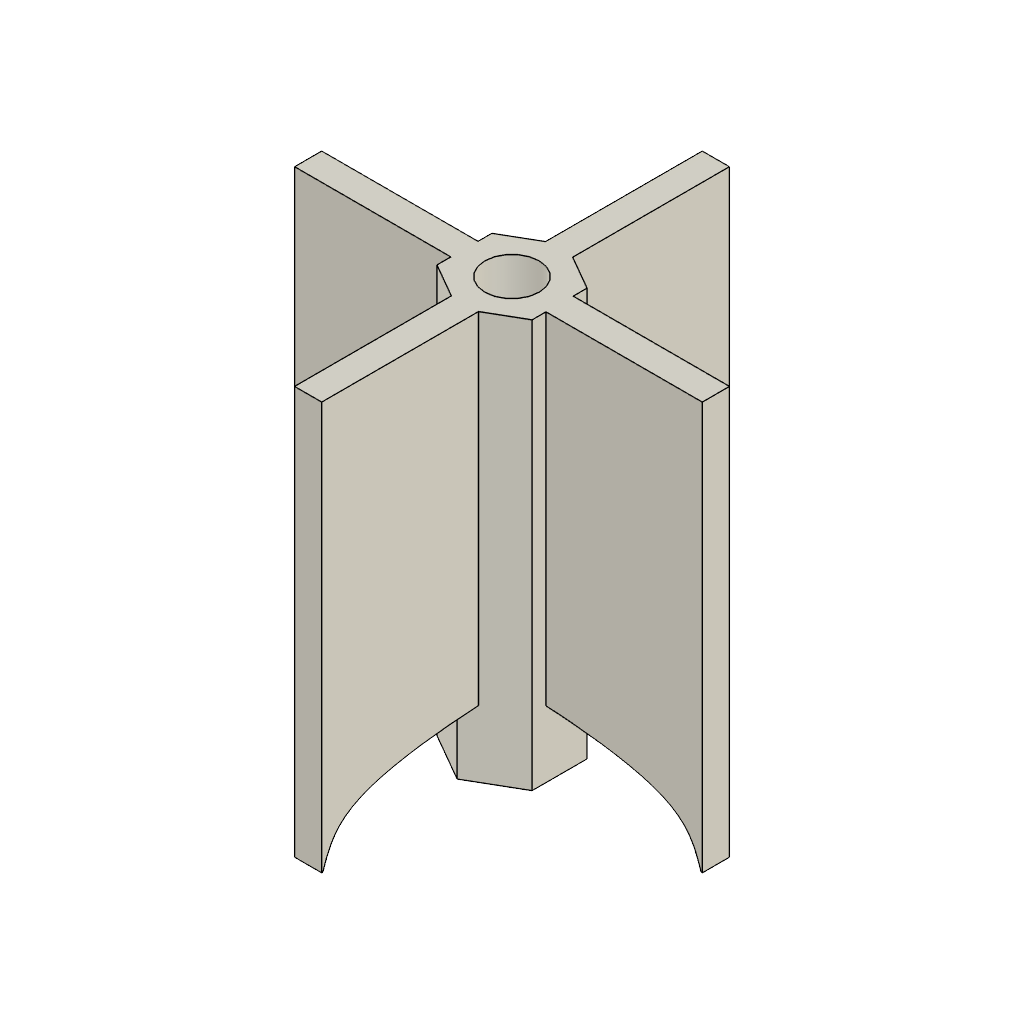
Sensor Assembly (Autodesk Fusion 360 archive; units mm, degrees)
design "Sensor Divider 3 cm"
part number: 2026-09-18-10-50-11-663
Autodesk Fusion 360 part; units mm, degrees
sketch "Sketch1" plane through (0, 0, 0) normal (0, 0, 1) x (1, 0, 0)
  line L0 (-15, 0) -> (15, 0)
  line L1 (0, -15) -> (0, 15)
  line L2 (1, 15) -> (-1, 15)
  line L3 (-1, 15) -> (-1, -15)
  line L4 (-1, -15) -> (1, -15)
  line L5 (1, -15) -> (1, 15)
  line L6 (1, 15) -> (-1, -15) construction
  line L7 (-1, 15) -> (1, -15) construction
  line L8 (15, -1) -> (-15, -1)
  line L9 (-15, -1) -> (-15, 1)
  line L10 (-15, 1) -> (15, 1)
  line L11 (15, 1) -> (15, -1)
  line L12 (15, -1) -> (-15, 1) construction
  line L13 (-15, -1) -> (15, 1) construction
  line L14 (3.5, 2.25) -> (3.5, -2.25)
  line L15 (-0.1986, -4.1561) -> (3.6986, -1.9061)
  line L16 (0.1986, -4.1561) -> (-3.6986, -1.9061)
  line L17 (-3.6986, 1.9061) -> (0.1986, 4.1561)
  line L18 (3.6986, 1.9061) -> (-0.1986, 4.1561)
  line L19 (-3.5, 2.25) -> (-3.5, -2.25)
  circle A0 centre (0, 0) radius 2
  dimension "d1" = 30
  dimension "d2" = 30
  dimension "d3" = 4.5
  dimension "d4" = 4.5
  dimension "d5" = 4
  constraint midpoint L0 A0.centre
  constraint coincident A0.centre origin
  constraint horizontal L0
  constraint midpoint L1 A0.centre
  constraint perpendicular L0 L1
  constraint horizontal L2
  constraint perpendicular L2 L3
  constraint parallel L2 L4
  constraint parallel L3 L5
  constraint coincident L6 A0.centre
  constraint coincident L7 A0.centre
  constraint horizontal L8
  constraint perpendicular L8 L9
  constraint parallel L8 L10
  constraint parallel L9 L11
  constraint coincident L12 A0.centre
  constraint coincident L13 A0.centre
  measures "d1" distance of L0.start L0.end
  measures "d2" distance of L1.start L1.end
  measures "d3" distance of L14.start L14.end
  measures "d4" distance of L19.start L19.end
  measures "d5" diameter of A0
extrude "Extrude1" add sketch "Sketch1" along normal blind 30 contours L0 L9 L10 L19 | L0 L8 L9 L19 | L0 L10 L19 A0 | L0 L8 L19 A0 | L3 L10 L17 L19 A0 | L3 L8 L16 L19 A0 | L1 L3 L17 A0 | L1 L3 L16 A0 | L1 L2 L3 L17 | L1 L3 L4 L16 | L1 L5 L18 A0 | L1 L5 L15 A0 | L1 L2 L5 L18 | L1 L4 L5 L15 | L0 L10 L14 A0 | L0 L8 L14 A0 | L5 L10 L14 L18 A0 | L5 L8 L14 L15 A0 | L0 L10 L11 L14 | L0 L8 L11 L14
sketch "Sketch2" plane through (0, 0, 0) normal (0, 1, 0) x (1, 0, 0)
  spline S0 degree 5 poles (1.976, -4.9412) (2.1036, -4.9412) (2.3816, -4.9392) (2.8674, -4.93) (3.6828, -4.9007) (5.1251, -4.8061) (7.0462, -4.6109) (9.3872, -4.2698) (11.6257, -3.7307) (13.1893, -2.974) (14.1339, -2.0321) (14.549, -1.1666) (14.7949, -0.4741) (14.9482, 0.0041) (15.0223, 0.2474) knots 0 0 0 0 0 0 0.1 0.2 0.3 0.4 0.5 0.6 0.7 0.8 0.9 1 1 1 1 1 1
  line L0 (1.3362, -4.9412) -> (2.6158, -4.9412)
  line L1 (7.3223, -4.6412) -> (11.7829, -3.7228)
  line L2 (14.6638, -0.9298) -> (15.3808, 1.4246)
  line L3 (15.0223, -4.9412) -> (15.0223, 0.2474)
  line L4 (1.976, -4.9412) -> (15.0223, -4.9412)
  line L5 (15.0223, 0.2474) -> (1.976, 0.2474)
  line L6 (1.976, 0.2474) -> (1.976, -4.9412)
  line L7 (0, 0) -> (0, -4)
  point P0 (9.5526, -4.182)
  constraint midpoint P0 L1
  constraint midpoint S0.end L2
  constraint midpoint S0.start L0
  constraint coincident L0.end L4
  constraint coincident L7.start origin
  constraint vertical L7
revolve "Revolve1" cut sketch "Sketch2" angle 360 about axis through (0, 0, 0) along (0, 0, 1) contours S0 L5 L6
sketch "Sketch3" plane through (0, 0, 0) normal (0, 0, 1) x (1, 0, 0)
  line L0 (3.6986, 1.9061) -> (-0.1986, 4.1561)
  line L1 (-0.1986, -4.1561) -> (3.6986, -1.9061)
  line L2 (0.1986, -4.1561) -> (-3.6986, -1.9061)
  line L3 (-3.6986, 1.9061) -> (0.1986, 4.1561)
  line L4 (-3.5, 2.25) -> (-3.5, -2.25)
  line L5 (3.5, 2.25) -> (3.5, -2.25)
  dimension "d9" = 4.5
  dimension "d10" = 4.5
  measures "d9" distance of L5.start L5.end
  measures "d10" distance of L4.start L4.end
sketch "Sketch4" plane through (0, 0, 0) normal (0, 0, 1) x (1, 0, 0)
extrude "Extrude2" add sketch "Sketch3" along normal blind 9.5
sketch "Sketch5" plane through (0, 0, 0) normal (0, 0, -1) x (1, 0, 0)
  line L0 (3.5, 2.0207) -> (0, 4.0415)
  line L1 (0, 4.0415) -> (-3.5, 2.0207)
  line L2 (-3.5, 2.0207) -> (-3.5, -2.0207)
  line L3 (-3.5, -2.0207) -> (0, -4.0415)
  line L4 (0, -4.0415) -> (3.5, -2.0207)
  line L5 (3.5, -2.0207) -> (3.5, 2.0207)
  circle A0 centre (0, 0) radius 2
  dimension "d13" = 4
  constraint coincident A0.centre origin
  measures "d13" diameter of A0
extrude "Extrude3" cut sketch "Sketch5" against normal blind 28.5 contours A0

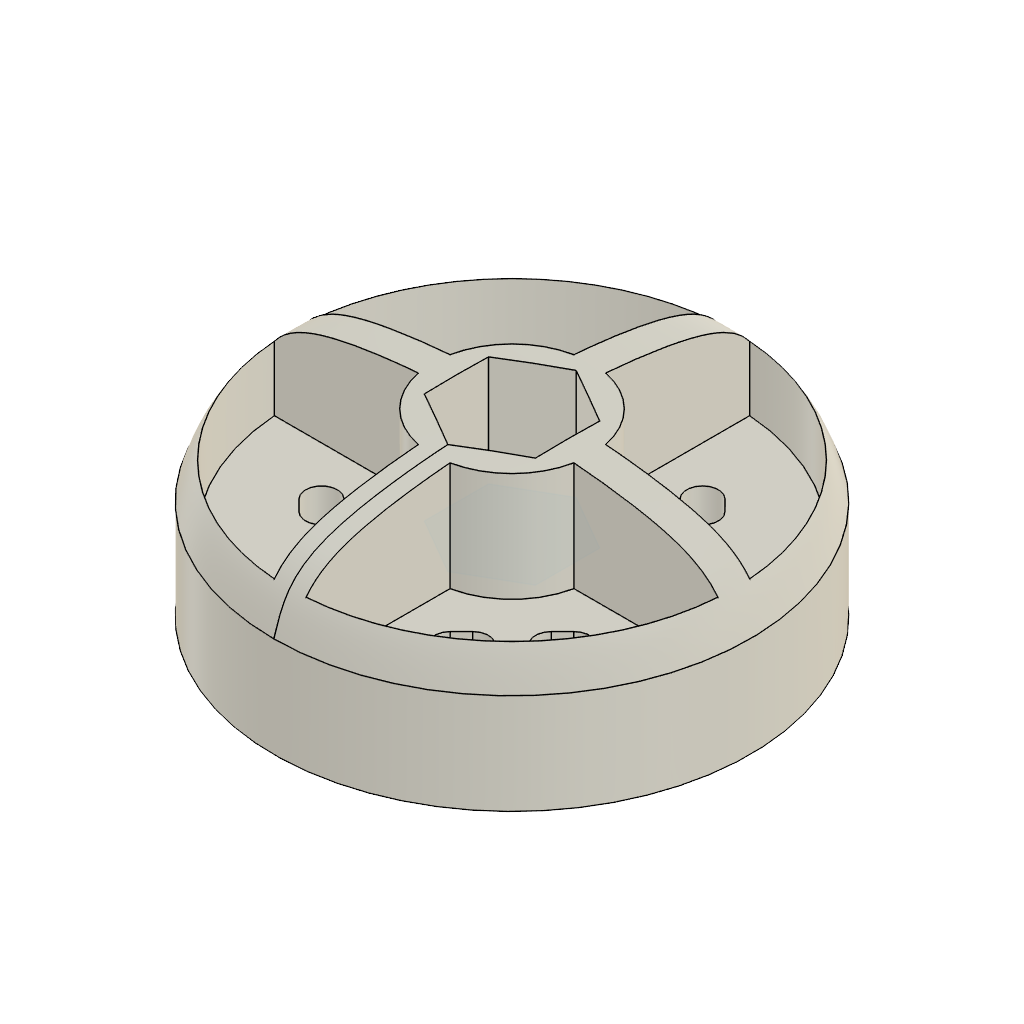
design "Sensor case Top V2"
part number: 2026-09-12-18-50-55-083
Autodesk Fusion 360 part; units mm, degrees
sketch "Sketch1" plane through (0, 0, 0) normal (0, 0, 1) x (1, 0, 0)
  circle A0 centre (0, 0) radius 15
  line L0 (-3.3472, 7.2366) -> (-4.0543, 6.5295)
  arc A1 (-3.3472, 7.2366) -> (-4.7617, 8.6505) centre (-4.0543, 7.9437) ccw
  arc A2 (-5.4683, 7.944) -> (-4.0543, 6.5295) centre (-4.7614, 7.2366) ccw
  line L1 (-4.7614, 8.6508) -> (-5.4685, 7.9437)
  arc A3 (-6.5292, 4.0546) -> (-7.963, 5.4487) centre (-7.2363, 4.7617) ccw
  line L2 (-7.963, 5.4487) -> (-8.6502, 4.762)
  arc A4 (-8.6502, 4.762) -> (-7.2363, 3.3475) centre (-7.9434, 4.0546) ccw
  line L3 (-6.5292, 4.0546) -> (-7.2363, 3.3475)
  line L4 (0, 15) -> (0, -15)
  line L5 (-15, 0) -> (15, 0)
  line L6 (0, 0) -> (-6, 6)
  line L7 (-4.7614, 7.2366) -> (-7.2363, 4.7617)
  circle A5 centre (-5.9989, 5.9992) radius 0.2772
  arc A6 (-7.944, -5.4683) -> (-6.5295, -4.0543) centre (-7.2366, -4.7614) ccw
  line L8 (-7.2366, -3.3472) -> (-6.5295, -4.0543)
  arc A7 (-7.2366, -3.3472) -> (-8.6505, -4.7617) centre (-7.9437, -4.0543) ccw
  line L9 (-8.6508, -4.7614) -> (-7.9437, -5.4685)
  arc A8 (-4.0546, -6.5292) -> (-5.4487, -7.963) centre (-4.7617, -7.2363) ccw
  line L10 (-5.4487, -7.963) -> (-4.762, -8.6502)
  arc A9 (-4.762, -8.6502) -> (-3.3475, -7.2363) centre (-4.0546, -7.9434) ccw
  line L11 (-4.0546, -6.5292) -> (-3.3475, -7.2363)
  arc A10 (5.4683, -7.944) -> (4.0543, -6.5295) centre (4.7614, -7.2366) ccw
  line L12 (3.3472, -7.2366) -> (4.0543, -6.5295)
  arc A11 (3.3472, -7.2366) -> (4.7617, -8.6505) centre (4.0543, -7.9437) ccw
  line L13 (4.7614, -8.6508) -> (5.4685, -7.9437)
  arc A12 (6.5292, -4.0546) -> (7.963, -5.4487) centre (7.2363, -4.7617) ccw
  line L14 (7.963, -5.4487) -> (8.6502, -4.762)
  arc A13 (8.6502, -4.762) -> (7.2363, -3.3475) centre (7.9434, -4.0546) ccw
  line L15 (6.5292, -4.0546) -> (7.2363, -3.3475)
  arc A14 (7.944, 5.4683) -> (6.5295, 4.0543) centre (7.2366, 4.7614) ccw
  line L16 (7.2366, 3.3472) -> (6.5295, 4.0543)
  arc A15 (7.2366, 3.3472) -> (8.6505, 4.7617) centre (7.9437, 4.0543) ccw
  line L17 (8.6508, 4.7614) -> (7.9437, 5.4685)
  arc A16 (4.0546, 6.5292) -> (5.4487, 7.963) centre (4.7617, 7.2363) ccw
  line L18 (5.4487, 7.963) -> (4.762, 8.6502)
  arc A17 (4.762, 8.6502) -> (3.3475, 7.2363) centre (4.0546, 7.9434) ccw
  line L19 (4.0546, 6.5292) -> (3.3475, 7.2363)
  dimension "d1" = 30
  dimension "d29" = 2
  dimension "d30" = 2
  dimension "d31" = 2
  dimension "d32" = 2
  dimension "d34" = 360
  constraint coincident A0.centre L6.start
  constraint coincident L2.end A4
  constraint tangent L2 A4
  constraint tangent A4 L3
  constraint coincident A4.start L2
  constraint coincident A1.end L1
  constraint coincident A2.start L1
  constraint coincident A0 L4.start
  constraint coincident A0 L4.end
  constraint perpendicular A0 L4
  constraint coincident A0 L5.start
  constraint coincident A0 L5.end
  constraint perpendicular A0 L5
  constraint coincident A2.centre L7.start
  constraint coincident A3.centre L7.end
  constraint midpoint L7 A5.centre
  measures "d1" diameter of A0
  measures "d29" diameter of A3
  measures "d30" diameter of A2
  measures "d31" diameter of A4
  measures "d32" diameter of A1
extrude "Extrude1" add sketch "Sketch1" along normal blind 4.5 contours A0 L4 L5 | A0 L4 L5 | A0 L4 L5 | A0 L4 L5 | L6 L7 A5 | L6 L7 A5 | L7 A5
sketch "Sketch2" plane through (0, 0, 4.5) normal (0, 0, 1) x (-1, 0, 0)
  circle A0 centre (0, 0) radius 15
  line L0 (8.6502, -4.762) -> (7.963, -5.4487)
  arc A1 (6.5292, -4.0546) -> (7.963, -5.4487) centre (7.2363, -4.7617) ccw
  line L1 (6.5292, -4.0546) -> (7.2363, -3.3475)
  arc A2 (8.6502, -4.762) -> (7.2363, -3.3475) centre (7.9434, -4.0546) ccw
  line L2 (-8.6502, 4.762) -> (-7.963, 5.4487)
  arc A3 (-6.5292, 4.0546) -> (-7.963, 5.4487) centre (-7.2363, 4.7617) ccw
  line L3 (-6.5292, 4.0546) -> (-7.2363, 3.3475)
  arc A4 (-8.6502, 4.762) -> (-7.2363, 3.3475) centre (-7.9434, 4.0546) ccw
  arc A5 (3.3472, -7.2366) -> (4.7614, -8.6508) centre (4.0543, -7.9437) ccw
  line L4 (3.3472, -7.2366) -> (4.0543, -6.5295)
  arc A6 (5.4685, -7.9437) -> (4.0543, -6.5295) centre (4.7614, -7.2366) ccw
  line L5 (5.4685, -7.9437) -> (4.7614, -8.6508)
  line L6 (-4.762, -8.6502) -> (-5.4487, -7.963)
  arc A7 (-4.0546, -6.5292) -> (-5.4487, -7.963) centre (-4.7617, -7.2363) ccw
  line L7 (-4.0546, -6.5292) -> (-3.3475, -7.2363)
  arc A8 (-4.762, -8.6502) -> (-3.3475, -7.2363) centre (-4.0546, -7.9434) ccw
  arc A9 (7.2366, 3.3472) -> (8.6508, 4.7614) centre (7.9437, 4.0543) ccw
  line L8 (7.2366, 3.3472) -> (6.5295, 4.0543)
  arc A10 (7.9437, 5.4685) -> (6.5295, 4.0543) centre (7.2366, 4.7614) ccw
  line L9 (7.9437, 5.4685) -> (8.6508, 4.7614)
  line L10 (4.762, 8.6502) -> (5.4487, 7.963)
  arc A11 (4.0546, 6.5292) -> (5.4487, 7.963) centre (4.7617, 7.2363) ccw
  line L11 (4.0546, 6.5292) -> (3.3475, 7.2363)
  arc A12 (4.762, 8.6502) -> (3.3475, 7.2363) centre (4.0546, 7.9434) ccw
  arc A13 (-7.2366, -3.3472) -> (-8.6508, -4.7614) centre (-7.9437, -4.0543) ccw
  line L12 (-7.2366, -3.3472) -> (-6.5295, -4.0543)
  arc A14 (-7.9437, -5.4685) -> (-6.5295, -4.0543) centre (-7.2366, -4.7614) ccw
  line L13 (-7.9437, -5.4685) -> (-8.6508, -4.7614)
  arc A15 (-3.3472, 7.2366) -> (-4.7614, 8.6508) centre (-4.0543, 7.9437) ccw
  line L14 (-3.3472, 7.2366) -> (-4.0543, 6.5295)
  arc A16 (-5.4685, 7.9437) -> (-4.0543, 6.5295) centre (-4.7614, 7.2366) ccw
  line L15 (-5.4685, 7.9437) -> (-4.7614, 8.6508)
  line L16 (0, 0) -> (0, -15)
  line L17 (0, 15) -> (0, 0)
  line L18 (15, 0) -> (-15, 0)
  circle A17 centre (0, 0) radius 14
  line L19 (-1, -15) -> (1, -15)
  line L20 (1, -15) -> (1, 15)
  line L21 (1, 15) -> (-1, 15)
  line L22 (-1, 15) -> (-1, -15)
  line L23 (-1, -15) -> (1, 15) construction
  line L24 (1, -15) -> (-1, 15) construction
  line L25 (-15, 1) -> (15, 1)
  line L26 (15, 1) -> (15, -1)
  line L27 (15, -1) -> (-15, -1)
  line L28 (-15, -1) -> (-15, 1)
  line L29 (-15, 1) -> (15, -1) construction
  line L30 (15, 1) -> (-15, -1) construction
  line L31 (3.5, 0) -> (-3.5, 0)
  circle A18 centre (6, -6) radius 2.5
  line L32 (3.5, 2.25) -> (3.5, -2.25)
  line L33 (-3.5, 2.25) -> (-3.5, -2.25)
  line L34 (-3.6986, 1.9061) -> (0.1986, 4.1561)
  line L35 (-0.1986, -4.1561) -> (3.6986, -1.9061)
  line L36 (0.1986, -4.1561) -> (-3.6986, -1.9061)
  line L37 (3.6986, 1.9061) -> (-0.1986, 4.1561)
  circle A19 centre (0, 0) radius 5
  dimension "d37" = 28
  dimension "d38" = 7
  dimension "d39" = 5
  dimension "d40" = 4.5
  dimension "d41" = 4.5
  dimension "d43" = 360
  dimension "d44" = 10
  constraint coincident A0.centre L16.start
  constraint coincident A0 L16.end
  constraint vertical L16
  constraint coincident A0 L17.start
  constraint parallel L16 L17
  constraint coincident A0 L18.start
  constraint coincident A0 L18.end
  constraint perpendicular A0 L18
  constraint horizontal L19
  constraint perpendicular L19 L20
  constraint parallel L19 L21
  constraint parallel L20 L22
  constraint coincident L23 A0.centre
  constraint coincident L24 A0.centre
  constraint horizontal L25
  constraint perpendicular L25 L26
  constraint parallel L25 L27
  constraint parallel L26 L28
  constraint coincident L29 A0.centre
  constraint coincident L30 A0.centre
  constraint midpoint A0.centre L31
  constraint perpendicular L16 L31
  constraint midpoint L31.start L32
  constraint perpendicular L27 L32
  constraint midpoint L31.end L33
  constraint perpendicular L27 L33
  measures "d37" diameter of A17
  measures "d38" distance of L31.start L31.end
  measures "d39" diameter of A18
  measures "d40" distance of L32.start L32.end
  measures "d41" distance of L33.start L33.end
  measures "d44" diameter of A19
extrude "Extrude2" add sketch "Sketch2" along normal blind 7 contours A0 L18 A17 L25 | A0 L18 A17 L27 | A0 A17 L20 L25 | A0 A17 L20 L27 | L18 A17 L27 A19 | L18 A17 L25 A19 | A0 L17 A17 L20 | A0 L16 A17 L20 | L18 L27 L32 A19 | L18 L25 L32 A19 | A0 L17 A17 L22 | L17 A17 L20 A19 | L20 L25 L32 L37 A19 | A0 L16 A17 L22 | L16 A17 L20 A19 | L20 L27 L32 L35 A19 | A0 A17 L22 L25 | L17 A17 L22 A19 | L17 L20 L37 A19 | A0 A17 L22 L27 | L16 A17 L22 A19 | L16 L20 L35 A19 | A0 L18 A17 L25 | L17 L22 L34 A19 | A0 L18 A17 L27 | L16 L22 L36 A19 | L18 A17 L25 A19 | L22 L25 L33 L34 A19 | L18 A17 L27 A19 | L22 L27 L33 L36 A19 | L18 L25 L33 A19 | L18 L27 L33 A19
sketch "Sketch3" plane through (0, 0, 0) normal (1, 0, 0) x (0, 1, 0)
  spline S0 degree 5 poles (-1.9536, 11.5) (-2.0813, 11.5) (-2.3593, 11.498) (-2.8451, 11.4888) (-3.6605, 11.4595) (-5.1028, 11.3649) (-7.0239, 11.1697) (-9.3649, 10.8286) (-11.6033, 10.2895) (-13.167, 9.5328) (-14.1116, 8.5909) (-14.5267, 7.7254) (-14.7726, 7.0329) (-14.9259, 6.5546) (-15, 6.3114) knots 0 0 0 0 0 0 0.1 0.2 0.3 0.4 0.5 0.6 0.7 0.8 0.9 1 1 1 1 1 1
  line L0 (-1.9536, 11.5) -> (-15, 11.5)
  line L1 (-15, 11.5) -> (-15, 6.3114)
  line L2 (-15, 6.3114) -> (-1.9536, 6.3114)
  line L3 (-1.9536, 6.3114) -> (-1.9536, 11.5)
  line L4 (-7.3, 11.2) -> (-11.7606, 10.2816)
  line L5 (-14.6415, 7.4886) -> (-15.3585, 5.1342)
  line L6 (0, 10) -> (0, 15)
  line L7 (-1.3138, 11.5) -> (-2.5934, 11.5)
  point P0 (-9.5303, 10.7408)
  constraint horizontal L0
  constraint vertical L1
  constraint horizontal L2
  constraint vertical L3
  constraint midpoint P0 L4
  constraint midpoint S0.end L5
  constraint vertical L6
  constraint midpoint S0.start L7
  constraint coincident L0 L7.end
revolve "Revolve1" cut sketch "Sketch3" angle 360 about axis through (0, 0, 10) along (0, 0, 1) contours S0 L0 L1 L7
sketch "Sketch4" plane through (0, 0, 4.5) normal (0, 0, 1) x (-1, 0, 0)
  line L0 (-3.5, -2.0207) -> (0, -4.0415)
  line L1 (0, -4.0415) -> (3.5, -2.0207)
  line L2 (3.5, -2.0207) -> (3.5, 2.0207)
  line L3 (3.5, 2.0207) -> (0, 4.0415)
  line L4 (0, 4.0415) -> (-3.5, 2.0207)
  line L5 (-3.5, 2.0207) -> (-3.5, -2.0207)
sketch "Sketch5" plane through (0, 0, 4.5) normal (0, 0, 1) x (-1, 0, 0)
  circle A0 centre (0, 0) radius 2
  dimension "d48" = 4
  constraint coincident A0.centre origin
  measures "d48" diameter of A0
extrude "Extrude3" cut sketch "Sketch5" against normal blind 17
sketch "Sketch6" plane through (0, 0, 4.5) normal (0, 0, 1) x (-1, 0, 0)
  line L0 (13.9642, -1) -> (4.899, -1)
  arc A0 (1, -4.899) -> (4.899, -1) centre (0, 0) ccw
  line L1 (1, -4.899) -> (1, -13.9642)
  arc A1 (1, -13.9642) -> (13.9642, -1) centre (0, 0) ccw
  arc A2 (3.3472, -7.2366) -> (4.7614, -8.6508) centre (4.0543, -7.9437) ccw
  line L2 (3.3472, -7.2366) -> (4.0543, -6.5295)
  arc A3 (5.4685, -7.9437) -> (4.0543, -6.5295) centre (4.7614, -7.2366) ccw
  line L3 (5.4685, -7.9437) -> (4.7614, -8.6508)
  line L4 (8.6502, -4.762) -> (7.963, -5.4487)
  arc A4 (6.5292, -4.0546) -> (7.963, -5.4487) centre (7.2363, -4.7617) ccw
  line L5 (6.5292, -4.0546) -> (7.2363, -3.3475)
  arc A5 (8.6502, -4.762) -> (7.2363, -3.3475) centre (7.9434, -4.0546) ccw
  line L6 (7.2363, -4.7617) -> (4.7614, -7.2366)
  line L7 (6.8082, -4.8211) -> (4.8333, -6.8263)
  line L8 (4.8333, -6.8263) -> (5.1895, -7.1772)
  line L9 (5.1895, -7.1772) -> (7.1645, -5.172)
  line L10 (7.1645, -5.172) -> (6.8082, -4.8211)
  line L11 (6.8082, -4.8211) -> (5.1895, -7.1772) construction
  line L12 (4.8333, -6.8263) -> (7.1645, -5.172) construction
  line L13 (6.8263, 4.8333) -> (7.1772, 5.1895)
  line L14 (7.1772, 5.1895) -> (5.172, 7.1645)
  line L15 (4.8211, 6.8082) -> (6.8263, 4.8333)
  line L16 (5.172, 7.1645) -> (4.8211, 6.8082)
  line L17 (-4.8333, 6.8263) -> (-5.1895, 7.1772)
  line L18 (-5.1895, 7.1772) -> (-7.1645, 5.172)
  line L19 (-6.8082, 4.8211) -> (-4.8333, 6.8263)
  line L20 (-7.1645, 5.172) -> (-6.8082, 4.8211)
  line L21 (-6.8263, -4.8333) -> (-7.1772, -5.1895)
  line L22 (-7.1772, -5.1895) -> (-5.172, -7.1645)
  line L23 (-4.8211, -6.8082) -> (-6.8263, -4.8333)
  line L24 (-5.172, -7.1645) -> (-4.8211, -6.8082)
  point P0 (5.9989, -5.9992)
  dimension "d51" = 0.5
  dimension "d53" = 360
  constraint coincident A4.centre L6.start
  constraint coincident A3.centre L6.end
  constraint perpendicular L7 L8
  constraint parallel L7 L9
  constraint parallel L8 L10
  constraint coincident L11 P0
  constraint coincident L12 P0
  constraint midpoint L6 P0
  measures "d51" distance of L7.end L8.end
extrude "Extrude4" cut sketch "Sketch6" against normal blind 3 contours A3 A4 L6 L7 | A3 A4 L6 L9 | L13 L14 L15 L16 | L17 L18 L19 L20 | L21 L22 L23 L24

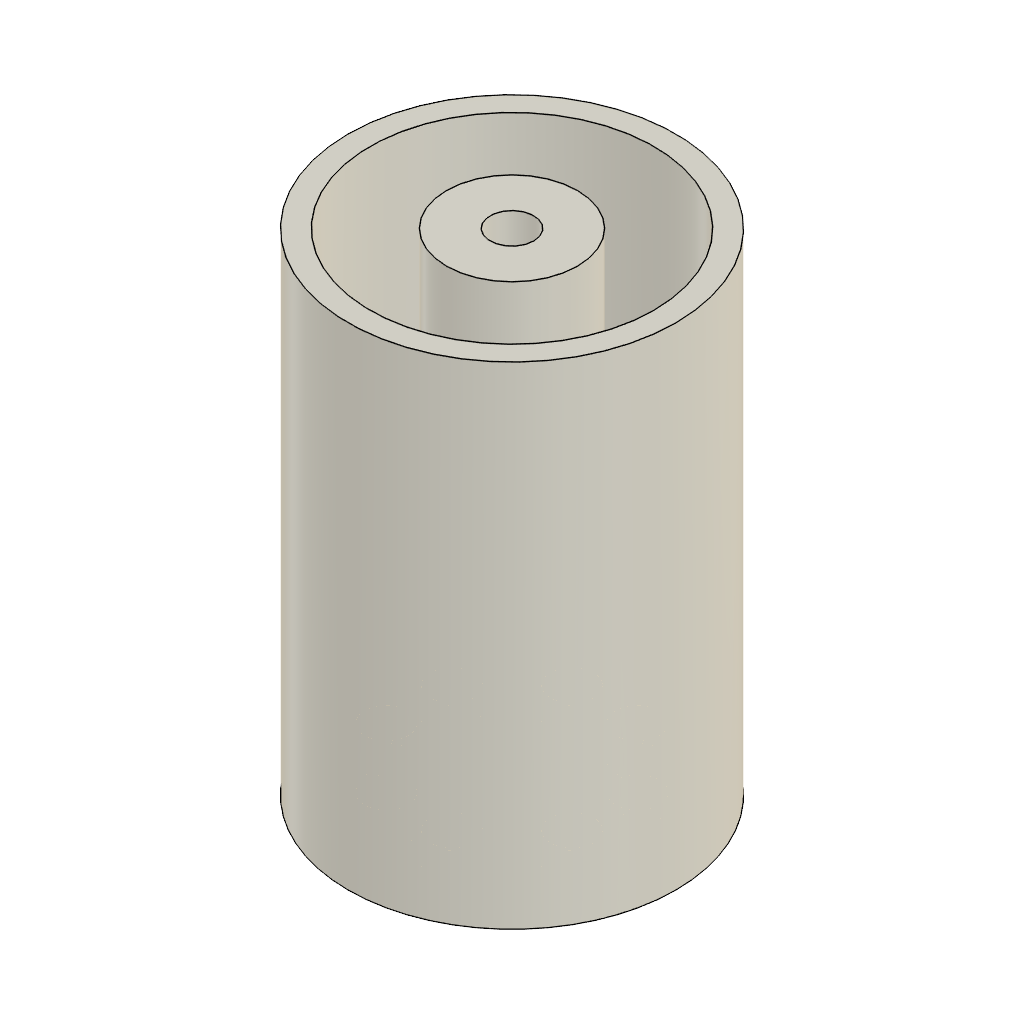
design "Sensor case Bottem"
part number: 2026-09-12-19-29-05-457
Autodesk Fusion 360 part; units mm, degrees
sketch "Sketch1" plane through (0, 0, 0) normal (0, 0, 1) x (1, 0, 0)
  circle A0 centre (0, 0) radius 15
  line L0 (0, 0) -> (0, 8.5)
  line L1 (0, 0) -> (0, -8.5)
  line L2 (0, -8.5) -> (0, 0)
  line L3 (0, 0) -> (-8.5, 0)
  line L4 (-8.5, 0) -> (0, 0)
  line L5 (0, 0) -> (8.5, 0)
  line L6 (-8.5, -1) -> (-8.5, 1)
  line L7 (1, 8.5) -> (-1, 8.5)
  line L8 (8.5, -1) -> (8.5, 1)
  line L9 (1, -8.5) -> (-1, -8.5)
  circle A1 centre (-3, -8.5) radius 2
  circle A2 centre (3, -8.5) radius 2
  circle A3 centre (8.5, -3) radius 2
  circle A4 centre (8.5, 3) radius 2
  circle A5 centre (3, 8.5) radius 2
  circle A6 centre (-3, 8.5) radius 2
  circle A7 centre (-8.5, 3) radius 2
  circle A8 centre (-8.5, -3) radius 2
  dimension "d1" = 30
  dimension "d2" = 8.5
  dimension "d3" = 8.5
  dimension "d4" = 8.5
  dimension "d5" = 8.5
  dimension "d6" = 2
  dimension "d7" = 2
  dimension "d8" = 2
  dimension "d9" = 2
  dimension "d10" = 4
  dimension "d11" = 4
  dimension "d13" = 360
  constraint coincident A0.centre L0.start
  constraint vertical L0
  constraint parallel L0 L1
  constraint perpendicular L1 L3
  constraint perpendicular L2 L5
  constraint midpoint L3.end L6
  constraint perpendicular L4 L6
  constraint midpoint L0.end L7
  constraint perpendicular L0 L7
  constraint midpoint L5.end L8
  constraint perpendicular L5 L8
  constraint midpoint L1.end L9
  constraint perpendicular L1 L9
  constraint coincident L9.end A1
  constraint coincident L9.start A2
  measures "d1" diameter of A0
  measures "d2" distance of A0.centre L0.end
  measures "d3" distance of A0.centre L1.end
  measures "d4" distance of A0.centre L3.end
  measures "d5" distance of A0.centre L5.end
  measures "d6" distance of L6.start L6.end
  measures "d7" distance of L7.start L7.end
  measures "d8" distance of L8.start L8.end
  measures "d9" distance of L9.start L9.end
  measures "d10" diameter of A1
  measures "d11" diameter of A2
extrude "Extrude1" add sketch "Sketch1" along normal blind 3
sketch "Sketch2" plane through (0, 0, 3) normal (0, 0, 1) x (-1, 0, 0)
  circle A0 centre (0, 0) radius 15
  circle A1 centre (-3, -8.5) radius 2
  circle A2 centre (8.5, 3) radius 2
  circle A3 centre (3, -8.5) radius 2
  circle A4 centre (-8.5, -3) radius 2
  circle A5 centre (-8.5, 3) radius 2
  circle A6 centre (8.5, -3) radius 2
  circle A7 centre (-3, 8.5) radius 2
  circle A8 centre (3, 8.5) radius 2
  circle A9 centre (0, 0) radius 4
  circle A10 centre (0, 0) radius 6
  circle A11 centre (0, 0) radius 15
  circle A12 centre (0, 0) radius 13
  dimension "d16" = 8
  constraint coincident A0.centre A9.centre
  constraint concentric A9 A10
  constraint concentric A9 A11
  constraint concentric A10 A12
  measures "d16" diameter of A9
extrude "Extrude2" add sketch "Sketch2" along normal blind 42 contours A0 A11 | A10
sketch "Sketch3" plane through (0, 0, 3) normal (0, 0, 1) x (-1, 0, 0)
  circle A0 centre (0, 0) radius 4
  circle A1 centre (0, 0) radius 4
  constraint coincident A0.centre A1.centre
extrude "Extrude3" cut sketch "Sketch3" against normal blind 21
sketch "Sketch4" plane through (0, 0, 45) normal (0, 0, 1) x (-1, 0, 0)
  circle A0 centre (0, 0) radius 4
  circle A1 centre (0, 0) radius 6
  circle A2 centre (0, 0) radius 5
  circle A3 centre (0, 0) radius 2
  constraint coincident A0.centre A1.centre
extrude "Extrude4" add sketch "Sketch4" against normal blind 4 contours A0
